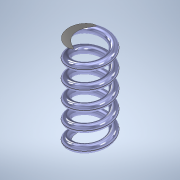
# Autodesk Inventor part: Part3
Saved by Autodesk Inventor 2020 (Build 240168000, 168)
## iProperties
Created: 2021-05-18
Part Number: Part3
Material: Steel, Carbon
Document SubType Name: Modeling
Designer: Andrew
Density: 7.85 g/cm^3
Appearance: Semi-Polished
Mass: 870.103 g
Surface Area: 372.006 cm^2
Volume: 110.841 cm^3
Author: Andrew
Autodesk Inventor part; units mm, degrees
ref_plane "YZ Plane" through (0, 0, 0) normal (1, 0, 0) x (0, 1, 0)
ref_plane "XZ Plane" through (0, 0, 0) normal (0, 1, 0) x (-1, 0, 0)
ref_plane "XY Plane" through (0, 0, 0) normal (0, 0, 1) x (1, 0, 0)
sketch "Sketch1" plane through (0, 0, 0) normal (0, 1, 0) x (-1, 0, 0)
  circle A0 centre (0, 0) radius 35
  dimension "d0" = 70
  constraints: 1 centre point, 1 coincident
  measures "d0" diameter of A0
extrude "Extrusion1" add sketch "Sketch1" along normal blind 150
sketch "Sketch2" plane through (0, 0, 0) normal (1, 0, 0) x (0, 1, 0)
  circle A0 centre (156.25, 28.755) radius 6.25
  line L0 (0, -35) -> (0, 35) projected
  line L1 (0, 0) -> (150, 0)
  line L2 (150, -35) -> (150, 35) projected
  dimension "d3" = 12.5
  dimension "d6" = 156.25
  dimension "d15" = 57.51
  constraints: 2 end point, 1 centre point, 1 midpoint
  measures "d3" diameter of A0
  measures "d6" distance from line of L0 A0.centre
  measures "d15" diameter of A0.centre L1
coil "Coil1" sketch "Sketch2" operation intersect axis through (0, 0, 0) along (0, -1, 0) pitch 30 turns 5.833333 hand right
body "Solid1"
